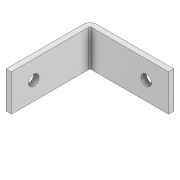
# Autodesk Inventor part: esquina de bandeja
Saved by Autodesk Inventor 2020.3 (Build 243373000, 373)
## iProperties
Created: 2020-06-07
Part Number: esquina de bandeja
Material: Aluminum 1100-H14
Document SubType Name: Modeling
Designer: Pipi
Density: 2.7 g/cm^3
Appearance: Satin
Author: Pipi
Autodesk Inventor part; units mm, degrees
ref_plane "YZ Plane" through (0, 0, 0) normal (1, 0, 0) x (0, 1, 0)
ref_plane "XZ Plane" through (0, 0, 0) normal (0, 1, 0) x (-1, 0, 0)
ref_plane "XY Plane" through (0, 0, 0) normal (0, 0, 1) x (1, 0, 0)
sketch "Boceto1" plane through (0, 0, 0) normal (0, 1, 0) x (-1, 0, 0)
  line L0 (-7.5247, -31.1664) -> (-7.5247, 0.8336)
  line L1 (-7.5247, 0.8336) -> (-9.5247, 0.8336)
  line L2 (-9.5247, 0.8336) -> (-9.5247, -29.1664)
  line L3 (-7.5247, -31.1664) -> (-39.5247, -31.1664)
  line L4 (-39.5247, -31.1664) -> (-39.5247, -29.1664)
  line L5 (-39.5247, -29.1664) -> (-9.5247, -29.1664)
  dimension "d46" = 32
  dimension "d47" = 2
  dimension "d48" = 30
  dimension "d49" = 32
  constraints: 12 end point, 4 perpendicular, 1 horizontal, 1 vertical
  measures "d46" distance of L0.start L0.end
  measures "d47" distance of L0.end L1.end
  measures "d48" distance of L1.end L2.end
  measures "d49" distance of L0.start L3.end
extrude "Extrusion9" add sketch "Boceto1" along normal blind 14
fillet "Fillet1" radius 0.5 1 edges at (9.5247, 7, -29.1664)
fillet "Fillet2" radius 2.5 1 edges at (7.5247, 7, -31.1664)
sketch "Sketch6" plane through (9.5247, 0, 0.8336) normal (1, 0, 0) x (0, 0, -1)
  circle A0 centre (8.5, 7) radius 2
  line L0 (30, 0) -> (30, 14) projected
  line L1 (0, 0) -> (29.5, 0) projected
  dimension "d54" = 4
  dimension "d55" = 21.5
  dimension "d56" = 7
  constraints: 1 centre point
  measures "d54" diameter of A0
  measures "d55" distance from line of A0.centre L0
  measures "d56" distance from line of L1 A0.centre
sketch "Sketch7" plane through (39.5247, 0, -29.1664) normal (0, 0, 1) x (1, 0, 0)
  circle A0 centre (-8.5, 7) radius 2
  line L0 (-29.5, 0) -> (0, 0) projected
  line L1 (-30, 14) -> (-30, 0) projected
  dimension "d57" = 4
  dimension "d58" = 7
  dimension "d59" = 21.5
  constraints: 1 centre point
  measures "d57" diameter of A0
  measures "d58" distance from line of L0 A0.centre
  measures "d59" distance from line of L1 A0.centre
extrude "Extrusion10" cut sketch "Sketch6" against normal blind 10
extrude "Extrusion11" cut sketch "Sketch7" against normal blind 10
body "Solid3"
